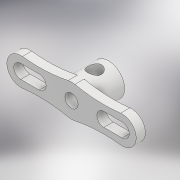
# Autodesk Inventor part: EncoderWheelAdapterSmallSlotted
Saved by Autodesk Inventor 2018.2 (Build 222227000, 227)
## iProperties
Created: 2018-03-25
Part Number: EncoderWheelAdapterSmallSlotted
Material: ABS Plastic
Document SubType Name: Modeling
Designer: mansu
Density: 1.06 g/cm^3
Appearance: Smooth - White
Mass: 0.492256 g
Surface Area: 7.06553 cm^2
Volume: 0.464392 cm^3
Author: mansu
Autodesk Inventor part; units mm, degrees
ref_plane "YZ Plane" through (0, 0, 0) normal (1, 0, 0) x (0, 1, 0)
ref_plane "XZ Plane" through (0, 0, 0) normal (0, 1, 0) x (-1, 0, 0)
sketch "Sketch1" plane through (0, 0, 0) normal (0, 1, 0) x (-1, 0, 0)
  circle A0 centre (0, 0) radius 1.425
  arc A1 (0.7325, 3.4225) -> (0.7325, -3.4225) centre (0, 0) ccw
  arc A2 (-10.6374, 2.978) -> (-10.6374, -2.978) centre (-11, 0) ccw
  arc A3 (-0.7325, -3.4225) -> (-10.6374, -2.978) centre (-7.0114, -32.7581) ccw
  arc A4 (-10.6374, 2.978) -> (-0.7325, 3.4225) centre (-7.0114, 32.7581) ccw
  line L0 (0, 0) -> (0, -3.5) construction
  arc A5 (10.6374, -2.978) -> (10.6374, 2.978) centre (11, 0) ccw
  arc A6 (10.6374, -2.978) -> (0.7325, -3.4225) centre (7.0114, -32.7581) ccw
  arc A7 (0.7325, 3.4225) -> (10.6374, 2.978) centre (7.0114, 32.7581) ccw
  arc A8 (0.7325, -3.4225) -> (0.7325, 3.4225) centre (0, 0) ccw
  line L1 (-7, 0) -> (-11, 0) construction
  line L2 (-7, 1.5) -> (-11, 1.5)
  line L3 (-11, -1.5) -> (-7, -1.5)
  arc A9 (-7, -1.5) -> (-7, 1.5) centre (-7, 0) ccw
  arc A10 (-11, 1.5) -> (-11, -1.5) centre (-11, 0) ccw
  line L4 (0, 0) -> (0, 10.6899) construction
  line L5 (7, 1.5) -> (11, 1.5)
  line L6 (11, -1.5) -> (7, -1.5)
  arc A11 (7, 1.5) -> (7, -1.5) centre (7, 0) ccw
  arc A12 (11, -1.5) -> (11, 1.5) centre (11, 0) ccw
  point P0 (-9, 0)
  dimension "d0" = 2.85
  dimension "d1" = 7
  dimension "d6" = 3
  dimension "d14" = 30
  dimension "d15" = 3
  dimension "d16" = 4
  dimension "d17" = 7
  constraints: 27 point on circle, 16 end point, 13 centre point, 13 symmetric about line, 8 tangent, 3 coincident, 2 vertical, 1 equal radius, 1 horizontal, 1 horizontal alignment, 1 midpoint, 1 parallel, 5 other
  measures "d0" diameter of A0
  measures "d1" diameter of A1
  measures "d6" radius of A2
  measures "d14" radius of A4
  measures "d15" diameter of A10
  measures "d16" distance of L1.start L1.end
  measures "d17" distance of point (0, 0) L1.start
extrude "Extrusion1" add sketch "Sketch1" against normal blind 2
extrude "Extrusion2" add sketch "Sketch1" along normal blind 6 contours A8 A1
sketch "Sketch2" plane through (0, 0, 0) normal (0, 0, 1) x (1, 0, 0)
  circle A0 centre (0, 3) radius 1.5
  line L0 (3.5, 6) -> (3.5, 0) projected
  point P0 (0, 0)
  point P1 (3.5, 3)
  dimension "d11" = 3
  constraints: 1 centre point, 1 horizontal alignment, 1 midpoint, 1 vertical alignment
  measures "d11" diameter of A0
extrude "Extrusion3" cut sketch "Sketch2" along normal through all both and the other way through all
ref_plane "Work Plane1" through (0, 0, 3.5) normal (0, 0, 1) x (1, 0, 0)
body "Solid1"
